Autodesk Fusion 360 part; units mm, degrees
note: some values were not read from the file. Set by a fixed rule: the direction of a hole.
(part 6 of 6)
  line L835 (112.245, -64.0081) -> (112.482, -64.0649)
  line L836 (112.482, -64.0649) -> (112.707, -64.1579)
  line L837 (112.707, -64.1579) -> (112.914, -64.285)
  line L838 (112.914, -64.285) -> (113.099, -64.443)
  line L839 (113.099, -64.443) -> (113.257, -64.6279)
  line L840 (113.257, -64.6279) -> (113.384, -64.8353)
  line L841 (113.384, -64.8353) -> (113.477, -65.06)
  line L842 (113.477, -65.06) -> (113.534, -65.2965)
  line L843 (113.534, -65.2965) -> (113.553, -65.539)
  line L844 (113.553, -65.539) -> (113.534, -65.7815)
  line L845 (113.534, -65.7815) -> (113.477, -66.018)
  line L846 (113.477, -66.018) -> (113.384, -66.2427)
  line L847 (113.384, -66.2427) -> (113.257, -66.4501)
  line L848 (113.257, -66.4501) -> (113.099, -66.635)
  line L849 (113.099, -66.635) -> (112.914, -66.793)
  line L850 (112.914, -66.793) -> (112.707, -66.9201)
  line L851 (112.707, -66.9201) -> (112.482, -67.0131)
  line L852 (112.482, -67.0131) -> (112.245, -67.0699)
  line L853 (112.245, -67.0699) -> (112.003, -67.089)
  line L854 (112.003, -67.089) -> (111.761, -67.0699)
  line L855 (111.761, -67.0699) -> (111.524, -67.0131)
  line L856 (111.524, -67.0131) -> (111.299, -66.9201)
  line L857 (111.299, -66.9201) -> (111.092, -66.793)
  line L858 (111.092, -66.793) -> (110.907, -66.635)
  line L859 (110.907, -66.635) -> (110.749, -66.4501)
  line L860 (110.749, -66.4501) -> (110.622, -66.2427)
  line L861 (110.622, -66.2427) -> (110.529, -66.018)
  line L862 (110.529, -66.018) -> (110.472, -65.7815)
  line L863 (110.472, -65.7815) -> (110.453, -65.539)
  line L864 (110.453, -65.539) -> (110.456, -65.5035)
  line L865 (110.456, -65.5035) -> (110.472, -65.2965)
  line L866 (110.472, -65.2965) -> (110.529, -65.06)
  line L867 (110.615, -65.9741) -> (110.704, -66.195)
  line L868 (110.704, -66.195) -> (110.829, -66.3983)
  line L869 (110.829, -66.3983) -> (110.985, -66.5785)
  line L870 (110.985, -66.5785) -> (111.168, -66.7308)
  line L871 (111.168, -66.7308) -> (111.374, -66.8511)
  line L872 (111.374, -66.8511) -> (111.597, -66.9362)
  line L873 (111.597, -66.9362) -> (111.831, -66.9837)
  line L874 (111.831, -66.9837) -> (112.069, -66.9925)
  line L875 (112.069, -66.9925) -> (112.306, -66.9622)
  line L876 (112.306, -66.9622) -> (112.534, -66.8937)
  line L877 (112.534, -66.8937) -> (112.748, -66.7888)
  line L878 (112.748, -66.7888) -> (112.942, -66.6503)
  line L879 (112.942, -66.6503) -> (113.111, -66.482)
  line L880 (113.111, -66.482) -> (113.25, -66.2884)
  line L881 (113.25, -66.2884) -> (113.356, -66.0746)
  line L882 (113.356, -66.0746) -> (113.425, -65.8465)
  line L883 (113.425, -65.8465) -> (113.456, -65.6101)
  line L884 (113.456, -65.6101) -> (113.458, -65.539)
  line L885 (113.458, -65.539) -> (113.438, -65.3014)
  line L886 (113.438, -65.3014) -> (113.38, -65.0701)
  line L887 (113.38, -65.0701) -> (113.285, -64.8515)
  line L888 (113.285, -64.8515) -> (113.156, -64.6513)
  line L889 (113.156, -64.6513) -> (112.995, -64.4749)
  line L890 (112.995, -64.4749) -> (112.808, -64.3271)
  line L891 (112.808, -64.3271) -> (112.599, -64.2119)
  line L892 (112.599, -64.2119) -> (112.375, -64.1323)
  line L893 (112.375, -64.1323) -> (112.14, -64.0905)
  line L894 (112.14, -64.0905) -> (111.902, -64.0876)
  line L895 (111.902, -64.0876) -> (111.666, -64.1236)
  line L896 (111.666, -64.1236) -> (111.439, -64.1977)
  line L897 (111.439, -64.1977) -> (111.228, -64.3078)
  line L898 (111.228, -64.3078) -> (111.037, -64.451)
  line L899 (111.037, -64.451) -> (110.872, -64.6234)
  line L900 (110.872, -64.6234) -> (110.738, -64.8203)
  line L901 (110.738, -64.8203) -> (110.638, -65.0366)
  line L902 (110.638, -65.0366) -> (110.574, -65.2664)
  line L903 (110.574, -65.2664) -> (110.548, -65.5035)
  line L904 (110.548, -65.5035) -> (110.562, -65.7415)
  line L905 (110.562, -65.7415) -> (110.615, -65.9741)
  line L906 (39.4089, -65.06) -> (39.5019, -64.8353)
  line L907 (39.5019, -64.8353) -> (39.629, -64.6279)
  line L908 (39.629, -64.6279) -> (39.787, -64.443)
  line L909 (39.787, -64.443) -> (39.9719, -64.285)
  line L910 (39.9719, -64.285) -> (40.1793, -64.1579)
  line L911 (40.1793, -64.1579) -> (40.404, -64.0649)
  line L912 (40.404, -64.0649) -> (40.6405, -64.0081)
  line L913 (40.6405, -64.0081) -> (40.883, -63.989)
  line L914 (40.883, -63.989) -> (41.1255, -64.0081)
  line L915 (41.1255, -64.0081) -> (41.362, -64.0649)
  line L916 (41.362, -64.0649) -> (41.5867, -64.1579)
  line L917 (41.5867, -64.1579) -> (41.7941, -64.285)
  line L918 (41.7941, -64.285) -> (41.979, -64.443)
  line L919 (41.979, -64.443) -> (42.137, -64.6279)
  line L920 (42.137, -64.6279) -> (42.2641, -64.8353)
  line L921 (42.2641, -64.8353) -> (42.3571, -65.06)
  line L922 (42.3571, -65.06) -> (42.4139, -65.2965)
  line L923 (42.4139, -65.2965) -> (42.433, -65.539)
  line L924 (42.433, -65.539) -> (42.4139, -65.7815)
  line L925 (42.4139, -65.7815) -> (42.3571, -66.018)
  line L926 (42.3571, -66.018) -> (42.2641, -66.2427)
  line L927 (42.2641, -66.2427) -> (42.137, -66.4501)
  line L928 (42.137, -66.4501) -> (41.979, -66.635)
  line L929 (41.979, -66.635) -> (41.7941, -66.793)
  line L930 (41.7941, -66.793) -> (41.5867, -66.9201)
  line L931 (41.5867, -66.9201) -> (41.362, -67.0131)
  line L932 (41.362, -67.0131) -> (41.1255, -67.0699)
  line L933 (41.1255, -67.0699) -> (40.883, -67.089)
  line L934 (40.883, -67.089) -> (40.6405, -67.0699)
  line L935 (40.6405, -67.0699) -> (40.404, -67.0131)
  line L936 (40.404, -67.0131) -> (40.1793, -66.9201)
  line L937 (40.1793, -66.9201) -> (39.9719, -66.793)
  line L938 (39.9719, -66.793) -> (39.787, -66.635)
  line L939 (39.787, -66.635) -> (39.629, -66.4501)
  line L940 (39.629, -66.4501) -> (39.5019, -66.2427)
  line L941 (39.5019, -66.2427) -> (39.4089, -66.018)
  line L942 (39.4089, -66.018) -> (39.3521, -65.7815)
  line L943 (39.3521, -65.7815) -> (39.333, -65.539)
  line L944 (39.333, -65.539) -> (39.3358, -65.5035)
  line L945 (39.3358, -65.5035) -> (39.3521, -65.2965)
  line L946 (39.3521, -65.2965) -> (39.4089, -65.06)
  line L947 (39.4946, -65.9741) -> (39.5843, -66.195)
  line L948 (39.5843, -66.195) -> (39.7089, -66.3983)
  line L949 (39.7089, -66.3983) -> (39.865, -66.5785)
  line L950 (39.865, -66.5785) -> (40.0485, -66.7308)
  line L951 (40.0485, -66.7308) -> (40.2543, -66.8511)
  line L952 (40.2543, -66.8511) -> (40.4771, -66.9362)
  line L953 (40.4771, -66.9362) -> (40.7107, -66.9837)
  line L954 (40.7107, -66.9837) -> (40.949, -66.9925)
  line L955 (40.949, -66.9925) -> (41.1855, -66.9622)
  line L956 (41.1855, -66.9622) -> (41.4139, -66.8937)
  line L957 (41.4139, -66.8937) -> (41.628, -66.7888)
  line L958 (41.628, -66.7888) -> (41.8221, -66.6503)
  line L959 (41.8221, -66.6503) -> (41.991, -66.482)
  line L960 (41.991, -66.482) -> (42.1302, -66.2884)
  line L961 (42.1302, -66.2884) -> (42.2358, -66.0746)
  line L962 (42.2358, -66.0746) -> (42.3051, -65.8465)
  line L963 (42.3051, -65.8465) -> (42.3362, -65.6101)
  line L964 (42.3362, -65.6101) -> (42.338, -65.539)
  line L965 (42.338, -65.539) -> (42.3184, -65.3014)
  line L966 (42.3184, -65.3014) -> (42.2603, -65.0701)
  line L967 (42.2603, -65.0701) -> (42.1653, -64.8515)
  line L968 (42.1653, -64.8515) -> (42.0358, -64.6513)
  line L969 (42.0358, -64.6513) -> (41.8753, -64.4749)
  line L970 (41.8753, -64.4749) -> (41.6882, -64.3271)
  line L971 (41.6882, -64.3271) -> (41.4794, -64.2119)
  line L972 (41.4794, -64.2119) -> (41.2547, -64.1323)
  line L973 (41.2547, -64.1323) -> (41.0199, -64.0905)
  line L974 (41.0199, -64.0905) -> (40.7815, -64.0876)
  line L975 (40.7815, -64.0876) -> (40.5458, -64.1236)
  line L976 (40.5458, -64.1236) -> (40.3192, -64.1977)
  line L977 (40.3192, -64.1977) -> (40.1077, -64.3078)
  line L978 (40.1077, -64.3078) -> (39.917, -64.451)
  line L979 (39.917, -64.451) -> (39.7523, -64.6234)
  line L980 (39.7523, -64.6234) -> (39.6179, -64.8203)
  line L981 (39.6179, -64.8203) -> (39.5175, -65.0366)
  line L982 (39.5175, -65.0366) -> (39.4538, -65.2664)
  line L983 (39.4538, -65.2664) -> (39.4285, -65.5035)
  line L984 (39.4285, -65.5035) -> (39.4422, -65.7415)
  line L985 (39.4422, -65.7415) -> (39.4946, -65.9741)
extrude "Extrude1" add sketch "SOLDERBREAD02_DXF_Outline_in_MilliMeters" along normal blind 2.54 contours L411 L412 L413 L414 L415 L416 L417 L418 L419 L420 L421 L422 L423 L424 L425 L426 L427 L428 L429 L430 L433 L434 L435 L436 L437 L440 L443 L444 L445 L446 L447 L450 L451 L452 L453 L454 L455 L456 L457 L458 L459 L460 L461 L462 L463 L464 L465 L466 L467 L468 L469 L470 L471 L472 L473 L474 L475 L476 L477 L478 L479 L480 L481 L482 L483 L484 L485 L486 L487 L488 L489 L490 L491 L492 L493 L494 L495 L496 L497 L498 L499 L500 L501 L502 L503 L504 L505 L506 L507 L508 L509 L510 L511 L512 L513 L514 L515 L516 L517 L518 L519 L520 L521 L523 L524 L525 L526 L527 L528 L529 L532 L533 L534 L535 L536 L537 L538 L539 L540 L541 L542 L543 L544 L545 L546 L547 L548 L549 L550 L551 L552 L553 L554 L555 L556 L557 L558 L559 L560 L561 L562 L563 L564 L565 L566 L567 L568 L569 L570 L571 L572 L573 L574 L575 L576 L577 L578 L579 L580 L581 L582 L583 L584 L585 L586 L587 L588 L589 L590 L591 L592 L593 L594 L595 L596 L599 L600 L601 L602 L603 L604 L605 L608 L609 L610 L611 L612 L616 L617 L618 L619 L620 L621 L622 L623 L624 L625 L626 L627 L628 L629 L630 L631 L632 L633 L634 L635 L636 L637 L638 L639 L640 L641 L642 L643 L644 L645 L646 L647 L648 L649 L650 L651 L652 L653 L654 L655 L656 L657 L658 L659 L660 L661 L662 L663 L664 L665 L666 L667 L668 L669 L670 L671 L672 L673 L674 L675 L676 L677 L678 L679 L680 L681 L682 L684 L685 L686 L687 L688 L689 L690 L691 L692 L693 L694 L695 L696 L697 L700 L701 L702 L703 L704 L705 L706 L707 L708 L709 L710 L711 L712 L713 L714 L715 L716 L717 L718 L719 L720 L721 L722 L723 L724 L725 L726 L727 L728 L729 L730 L731 L732 L733 L734 L735 L736 L737 L738 L739 L740 L741 L742 L743 L744 L745

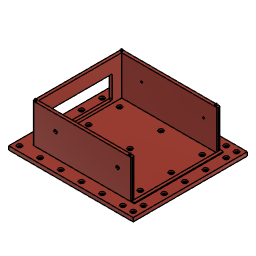
design "base"
Autodesk Fusion 360 part; units mm, degrees
sketch "Sketch1" plane through (0, 0, 0) normal (0, 0, 1) x (1, 0, 0)
  line L0 (0, 0) -> (232, 0)
  line L1 (232, 0) -> (232, 201)
  line L2 (232, 201) -> (0, 201)
  line L3 (0, 201) -> (0, 0)
  line L4 (0, 201) -> (-7, 201)
  line L5 (0, 201) -> (-7, 201)
  line L6 (-7, 201) -> (-7, 208)
  line L7 (-7, 208) -> (0, 208)
  line L8 (0, 208) -> (0, 201)
  line L9 (232, 0) -> (239, 0)
  line L10 (239, 0) -> (239, -7)
  line L11 (239, -7) -> (232, -7)
  line L12 (232, -7) -> (232, 0)
  line L13 (-7, 208) -> (239, 208)
  line L14 (239, 208) -> (239, -7)
  line L15 (239, -7) -> (-7, -7)
  line L16 (-7, -7) -> (-7, 208)
  line L17 (232, 201) -> (232, 208)
  line L18 (239, 208) -> (239, 240.3287)
  line L19 (-21.5407, 238.3287) -> (-21.5407, 225.3287)
  line L20 (-21.5407, 225.3287) -> (-34.5407, 225.3287)
  circle A0 centre (-21.5407, -24.6713) radius 5.75
  line L21 (266.4593, -37.6713) -> (253.4593, -37.6713)
  circle A1 centre (-21.5407, 25.3287) radius 3
  line L22 (253.4593, -37.6713) -> (253.4593, -24.6713)
  circle A2 centre (-21.5407, 225.3287) radius 5.75
  line L23 (-34.5407, 238.3287) -> (-21.5407, 238.3287)
  line L24 (-34.5407, 225.3287) -> (-34.5407, 238.3287)
  line L25 (253.4593, -24.6713) -> (266.4593, -24.6713)
  circle A3 centre (28.4593, -24.6713) radius 3
  circle A4 centre (-21.5407, 225.3287) radius 3
  circle A5 centre (253.4593, 0.3287) radius 5.75
  line L26 (266.4593, -24.6713) -> (266.4593, -37.6713)
  circle A6 centre (253.4593, -24.6713) radius 5.75
  circle A7 centre (-21.5407, 25.3287) radius 5.75
  circle A8 centre (253.4593, -24.6713) radius 3
  circle A9 centre (-21.5407, 75.3287) radius 3
  circle A10 centre (253.4593, 0.3287) radius 3
  circle A11 centre (253.4593, 50.3287) radius 5.75
  circle A12 centre (253.4593, 50.3287) radius 3
  circle A13 centre (128.4593, -24.6713) radius 5.75
  circle A14 centre (78.4593, -24.6713) radius 3
  circle A15 centre (28.4593, 225.3287) radius 3
  circle A16 centre (-21.5407, -24.6713) radius 3
  circle A17 centre (228.4593, -24.6713) radius 3
  circle A18 centre (78.4593, -24.6713) radius 5.75
  circle A19 centre (253.4593, 225.3287) radius 3
  circle A20 centre (253.4593, 225.3287) radius 5.75
  circle A21 centre (-21.5407, 175.3287) radius 3
  circle A22 centre (-21.5407, 125.3287) radius 3
  circle A23 centre (-21.5407, 125.3287) radius 5.75
  circle A24 centre (28.4593, -24.6713) radius 5.75
  circle A25 centre (-21.5407, 175.3287) radius 5.75
  line L27 (232.8, 201) -> (232.8, 208)
  circle A26 centre (78.4593, 225.3287) radius 3
  circle A27 centre (178.4593, 225.3287) radius 5.75
  circle A28 centre (128.4593, 225.3287) radius 5.75
  circle A29 centre (178.4593, 225.3287) radius 3
  circle A30 centre (178.4593, -24.6713) radius 3
  circle A31 centre (128.4593, -24.6713) radius 3
  circle A32 centre (28.4593, 225.3287) radius 5.75
  circle A33 centre (228.4593, 225.3287) radius 5.75
  circle A34 centre (253.4593, 200.3287) radius 3
  line L28 (266.4593, 238.3287) -> (266.4593, -37.6713)
  circle A35 centre (128.4593, 225.3287) radius 3
  circle A36 centre (-21.5407, 75.3287) radius 5.75
  circle A37 centre (228.4593, 225.3287) radius 3
  line L29 (266.4593, -37.6713) -> (-34.5407, -37.6713)
  line L30 (-34.5407, -37.6713) -> (-34.5407, 238.3287)
  circle A38 centre (228.4593, -24.6713) radius 5.75
  circle A39 centre (78.4593, 225.3287) radius 5.75
  circle A40 centre (178.4593, -24.6713) radius 5.75
  circle A41 centre (253.4593, 200.3287) radius 5.75
  line L31 (-34.5407, 238.3287) -> (266.4593, 238.3287)
  circle A42 centre (253.4593, 100.3287) radius 5.75
  circle A43 centre (253.4593, 150.3287) radius 3
  circle A44 centre (253.4593, 100.3287) radius 3
  circle A45 centre (253.4593, 150.3287) radius 5.75
  circle A46 centre (16, 180) radius 3.375
  circle A47 centre (16, 180) radius 5.75
  circle A48 centre (116, 180) radius 3.375
  circle A49 centre (116, 180) radius 5.75
  circle A50 centre (216, 180) radius 3.375
  circle A51 centre (216, 180) radius 5.75
  circle A52 centre (16, 105) radius 3.375
  circle A53 centre (16, 105) radius 5.75
  circle A54 centre (116, 105) radius 3.375
  circle A55 centre (116, 105) radius 5.75
  circle A56 centre (216, 105) radius 3.375
  circle A57 centre (216, 105) radius 5.75
  circle A58 centre (16, 30) radius 3.375
  circle A59 centre (16, 30) radius 5.75
  circle A60 centre (116, 30) radius 3.375
  circle A61 centre (116, 30) radius 5.75
  circle A62 centre (216, 30) radius 3.375
  circle A63 centre (216, 30) radius 5.75
  point P0 (0.8, 0)
  point P1 (0.8, 0)
  point P2 (0.8, 0)
  dimension "d2" = 201
  dimension "d3" = 7
  dimension "d4" = 7
  dimension "d5" = 7
  dimension "d6" = 7
  dimension "d56" = 7
  dimension "d156" = 25
  dimension "d157" = -25
  dimension "d160" = 25
  dimension "d161" = -25
  dimension "d162" = 11.5
  dimension "d163" = 6
  dimension "d164" = 13
  dimension "d165" = 13
  dimension "d166" = 13
  dimension "d167" = 13
  dimension "d168" = 7
  dimension "d223" = 6.75
  dimension "d224" = 11.5
  dimension "d227" = 100
  dimension "d228" = -75
  constraint vertical L1
  constraint horizontal L2
  constraint vertical L3
  constraint coincident L0.start L3.end
  constraint perpendicular L3 L4
  constraint horizontal L5
  constraint vertical L6
  constraint horizontal L7
  constraint vertical L8
  constraint horizontal L13
  constraint vertical L14
  constraint vertical L16
  constraint perpendicular L13 L17
  constraint concentric A2 A4
  constraint horizontal L20
  constraint vertical L24
  constraint horizontal L23
  constraint vertical L19
  constraint coincident L19.end L20.start
  constraint horizontal L25
  constraint vertical L26
  constraint horizontal L21
  constraint vertical L22
  constraint coincident L22.end L25.start
  constraint horizontal L29
  constraint vertical L30
  constraint horizontal L31
  constraint vertical L28
  constraint concentric A46 A47
  measures "d2" distance of L0.start L2.end
  measures "d3" distance of L2.end L4.end
  measures "d4" distance of L2.end L4.end
  measures "d5" distance of L2.end L7.end
  measures "d6" distance of L0.end L9.end
  measures "d56" distance of L1.end L17.end
  measures "d162" diameter of A2
  measures "d163" diameter of A4
  measures "d164" distance of L19.end L20.end
  measures "d165" distance of L19.end L19.start
  measures "d166" distance of L22.end L25.end
  measures "d167" distance of L22.end L21.end
  measures "d168" distance of L27.end L27.start
  measures "d223" diameter of A46
  measures "d224" diameter of A47
sketch "Sketch2" plane through (0, 0, 0) normal (0, 0, 1) x (1, 0, 0)
  circle A0 centre (-22.3407, 225.3287) radius 5.75
  circle A1 centre (27.6593, 225.3287) radius 5.75
  circle A2 centre (77.6593, 225.3287) radius 5.75
  circle A3 centre (127.6593, 225.3287) radius 5.75
  circle A4 centre (177.6593, 225.3287) radius 5.75
  circle A5 centre (227.6593, 225.3287) radius 5.75
  circle A6 centre (252.6593, 225.3287) radius 5.75
  circle A7 centre (252.6593, 200.3287) radius 5.75
  circle A8 centre (-22.3407, 175.3287) radius 5.75
  circle A9 centre (252.6593, 150.3287) radius 5.75
  circle A10 centre (-22.3407, 125.3287) radius 5.75
  circle A11 centre (252.6593, 100.3287) radius 5.75
  circle A12 centre (-22.3407, 75.3287) radius 5.75
  circle A13 centre (252.6593, 50.3287) radius 5.75
  circle A14 centre (-22.3407, 25.3287) radius 5.75
  circle A15 centre (252.6593, 0.3287) radius 5.75
  circle A16 centre (-22.3407, -24.6713) radius 5.75
  circle A17 centre (27.6593, -24.6713) radius 5.75
  circle A18 centre (77.6593, -24.6713) radius 5.75
  circle A19 centre (127.6593, -24.6713) radius 5.75
  circle A20 centre (177.6593, -24.6713) radius 5.75
  circle A21 centre (227.6593, -24.6713) radius 5.75
  circle A22 centre (252.6593, -24.6713) radius 5.75
  circle A23 centre (-22.3407, 225.3287) radius 3
  circle A24 centre (27.6593, 225.3287) radius 3
  circle A25 centre (77.6593, 225.3287) radius 3
  circle A26 centre (127.6593, 225.3287) radius 3
  circle A27 centre (177.6593, 225.3287) radius 3
  circle A28 centre (227.6593, 225.3287) radius 3
  circle A29 centre (252.6593, 225.3287) radius 3
  circle A30 centre (252.6593, 200.3287) radius 3
  circle A31 centre (-22.3407, 175.3287) radius 3
  circle A32 centre (252.6593, 150.3287) radius 3
  circle A33 centre (-22.3407, 125.3287) radius 3
  circle A34 centre (252.6593, 100.3287) radius 3
  circle A35 centre (-22.3407, 75.3287) radius 3
  circle A36 centre (252.6593, 50.3287) radius 3
  circle A37 centre (-22.3407, 25.3287) radius 3
  circle A38 centre (252.6593, 0.3287) radius 3
  circle A39 centre (-22.3407, -24.6713) radius 3
  circle A40 centre (27.6593, -24.6713) radius 3
  circle A41 centre (77.6593, -24.6713) radius 3
  circle A42 centre (127.6593, -24.6713) radius 3
  circle A43 centre (177.6593, -24.6713) radius 3
  circle A44 centre (227.6593, -24.6713) radius 3
  circle A45 centre (252.6593, -24.6713) radius 3
  line L0 (-22.3407, 225.3287) -> (-35.3407, 225.3287)
  line L1 (-35.3407, 225.3287) -> (-35.3407, 238.3287)
  line L2 (-35.3407, 238.3287) -> (-22.3407, 238.3287)
  line L3 (-22.3407, 238.3287) -> (-22.3407, 225.3287)
  line L4 (252.6593, -24.6713) -> (265.6593, -24.6713)
  line L5 (265.6593, -24.6713) -> (265.6593, -37.6713)
  line L6 (265.6593, -37.6713) -> (252.6593, -37.6713)
  line L7 (252.6593, -37.6713) -> (252.6593, -24.6713)
  line L8 (265.6593, -37.6713) -> (-35.3407, -37.6713)
  line L9 (-35.3407, -37.6713) -> (-35.3407, 238.3287)
  line L10 (-35.3407, 238.3287) -> (265.6593, 238.3287)
  line L11 (265.6593, 238.3287) -> (265.6593, -37.6713)
  line L12 (232, 201) -> (232, 208)
  dimension "d8" = 11.5
  dimension "d11" = 25
  dimension "d12" = -25
  dimension "d13" = 6
  dimension "d16" = 25
  dimension "d17" = -25
  dimension "d18" = 13
  dimension "d19" = 13
  dimension "d20" = 13
  dimension "d21" = 13
  dimension "d153" = 7
  constraint concentric A0 A23
  constraint horizontal L0
  constraint vertical L1
  constraint horizontal L2
  constraint vertical L3
  constraint coincident A0.centre A23.centre
  constraint horizontal L4
  constraint vertical L5
  constraint horizontal L6
  constraint vertical L7
  constraint coincident A22.centre A45.centre
  constraint horizontal L8
  constraint vertical L9
  constraint horizontal L10
  constraint vertical L11
  measures "d8" diameter of A0
  measures "d13" diameter of A23
  measures "d18" distance of A0.centre L0.end
  measures "d19" distance of A0.centre L2.end
  measures "d20" distance of A22.centre L4.end
  measures "d21" distance of A22.centre L6.end
  measures "d153" distance of L12.start L12.end
extrude "Extrude3" add sketch "Sketch1" along normal blind 7 contours L0 L1 L2 L3 | L0 L3 L4 L5 L12 L15 L16 | L1 L9 L13 L14 L17 | L9 L10 L11 L12 L14 L15 | L2 L8 L13 L17 | L4 L5 L6 L7 L8 L13 L16 makes body 1
extrude "Extrude4" add sketch "Sketch1" along normal blind 102 contours L0 L3 L4 L5 L12 L15 L16 | L2 L8 L13 L17 | L4 L5 L6 L7 L8 L13 L16 bodies 1
sketch "Sketch4" plane through (0, 0, 102) normal (0, 0, 1) x (-1, 0, 0)
  line L0 (0, -201) -> (-232, -201)
  line L1 (-232, -201) -> (-232, -208)
  line L2 (-232, -208) -> (7, -208)
  line L3 (7, -208) -> (7, 7)
  line L4 (7, 7) -> (-232, 7)
  line L5 (-232, 0) -> (0, 0)
  line L6 (0, 0) -> (0, -201)
  line L7 (7, -208) -> (-232, -208)
  line L8 (-232, -208) -> (-232, 0)
  line L9 (-232, 0) -> (7, 0)
  line L10 (7, 0) -> (7, -208)
  line L11 (-36, -158) -> (-198, -158)
  line L12 (-198, -158) -> (-198, -43)
  line L13 (-198, -43) -> (-36, -43)
  line L14 (-36, -43) -> (-36, -158)
  line L15 (7, -208) -> (-232, -208)
  line L16 (-232, -208) -> (-232, 7)
  line L17 (-232, 7) -> (7, 7)
  line L18 (7, 7) -> (7, -208)
  line L19 (-232, 7) -> (-225, 7)
  line L20 (-225, 7) -> (-225, 3.5)
  line L21 (-225, 3.5) -> (-232, 3.5)
  line L22 (-232, 3.5) -> (-232, 7)
  line L23 (7, 7) -> (3.5, 7)
  line L24 (3.5, 7) -> (3.5, 3.5)
  line L25 (3.5, 3.5) -> (7, 3.5)
  line L26 (7, 3.5) -> (7, 7)
  line L27 (7, -208) -> (3.5, -208)
  line L28 (3.5, -208) -> (3.5, -204.5)
  line L29 (3.5, -204.5) -> (7, -204.5)
  line L30 (7, -204.5) -> (7, -208)
  line L31 (-232, -208) -> (-225, -208)
  line L32 (-225, -208) -> (-225, -204.5)
  line L33 (-225, -204.5) -> (-232, -204.5)
  line L34 (-232, -204.5) -> (-232, -208)
  line L35 (1.625, -202.625) -> (5.375, -202.625)
  line L36 (5.375, -202.625) -> (5.375, -206.375)
  line L37 (5.375, -206.375) -> (1.625, -206.375)
  line L38 (1.625, -206.375) -> (1.625, -202.625)
  line L39 (1.625, -202.625) -> (5.375, -206.375) construction
  line L40 (5.375, -202.625) -> (1.625, -206.375) construction
  line L41 (1.625, 5.375) -> (5.375, 5.375)
  line L42 (5.375, 5.375) -> (5.375, 1.625)
  line L43 (5.375, 1.625) -> (1.625, 1.625)
  line L44 (1.625, 1.625) -> (1.625, 5.375)
  line L45 (1.625, 5.375) -> (5.375, 1.625) construction
  line L46 (5.375, 5.375) -> (1.625, 1.625) construction
  line L47 (-226.875, 5.375) -> (-223.125, 5.375)
  line L48 (-223.125, 5.375) -> (-223.125, 1.625)
  line L49 (-223.125, 1.625) -> (-226.875, 1.625)
  line L50 (-226.875, 1.625) -> (-226.875, 5.375)
  line L51 (-226.875, 5.375) -> (-223.125, 1.625) construction
  line L52 (-223.125, 5.375) -> (-226.875, 1.625) construction
  line L53 (-226.875, -202.625) -> (-223.125, -202.625)
  line L54 (-223.125, -202.625) -> (-223.125, -206.375)
  line L55 (-223.125, -206.375) -> (-226.875, -206.375)
  line L56 (-226.875, -206.375) -> (-226.875, -202.625)
  line L57 (-226.875, -202.625) -> (-223.125, -206.375) construction
  line L58 (-223.125, -202.625) -> (-226.875, -206.375) construction
  line L59 (-36, -158) -> (-15.2, -158)
  line L60 (-15.2, -158) -> (-15.2, -179.35)
  line L61 (-15.2, -179.35) -> (-36, -179.35)
  line L62 (-36, -179.35) -> (-36, -158)
  line L63 (-198, -43) -> (-218.8, -43)
  line L64 (-218.8, -43) -> (-218.8, -21.65)
  line L65 (-218.8, -21.65) -> (-198, -21.65)
  line L66 (-198, -21.65) -> (-198, -43)
  line L67 (-15.2, -179.35) -> (-218.8, -179.35)
  line L68 (-218.8, -179.35) -> (-218.8, -21.65)
  line L69 (-218.8, -21.65) -> (-15.2, -21.65)
  line L70 (-15.2, -21.65) -> (-15.2, -179.35)
  line L71 (-15.2, -179.35) -> (-10.2, -179.35)
  line L72 (-10.2, -179.35) -> (-10.2, -184.35)
  line L73 (-10.2, -184.35) -> (-15.2, -184.35)
  line L74 (-15.2, -184.35) -> (-15.2, -179.35)
  line L75 (-218.8, -21.65) -> (-223.8, -21.65)
  line L76 (-223.8, -21.65) -> (-223.8, -16.65)
  line L77 (-223.8, -16.65) -> (-218.8, -16.65)
  line L78 (-218.8, -16.65) -> (-218.8, -21.65)
  line L79 (-10.2, -184.35) -> (-223.8, -184.35)
  line L80 (-223.8, -184.35) -> (-223.8, -16.65)
  line L81 (-223.8, -16.65) -> (-10.2, -16.65)
  line L82 (-10.2, -16.65) -> (-10.2, -184.35)
  line L83 (-232, 7) -> (-232, 0)
  point P0 (3.5, -204.5)
  point P1 (3.5, 3.5)
  point P2 (-225, 3.5)
  point P3 (-225, -204.5)
  dimension "d59" = 162
  dimension "d60" = 115
  dimension "d89" = 7
  dimension "d90" = 3.5
  dimension "d91" = 3.5
  dimension "d92" = 3.5
  dimension "d93" = 3.5
  dimension "d94" = 3.5
  dimension "d95" = 7
  dimension "d96" = 3.75
  dimension "d97" = 3.75
  dimension "d98" = 3.75
  dimension "d99" = 3.75
  dimension "d100" = 3.75
  dimension "d101" = 3.75
  dimension "d102" = 3.75
  dimension "d103" = 3.75
  dimension "d104" = 20.8
  dimension "d105" = 21.35
  dimension "d106" = 20.8
  dimension "d107" = 21.35
  dimension "d108" = 5
  dimension "d109" = 5
  dimension "d110" = 5
  dimension "d111" = 5
  dimension "d112" = 3.5
  constraint horizontal L7
  constraint vertical L8
  constraint horizontal L9
  constraint vertical L10
  constraint coincident L5.start L8.end
  constraint coincident L2.end L3.start
  constraint horizontal L11
  constraint vertical L12
  constraint horizontal L13
  constraint vertical L14
  constraint horizontal L15
  constraint vertical L16
  constraint horizontal L17
  constraint vertical L18
  constraint coincident L4.end L16.end
  constraint horizontal L19
  constraint vertical L20
  constraint horizontal L21
  constraint vertical L22
  constraint horizontal L23
  constraint vertical L24
  constraint horizontal L25
  constraint vertical L26
  constraint coincident L3.end L4.start
  constraint horizontal L27
  constraint vertical L28
  constraint horizontal L29
  constraint vertical L30
  constraint horizontal L31
  constraint vertical L32
  constraint horizontal L33
  constraint vertical L34
  constraint horizontal L35
  constraint perpendicular L35 L36
  constraint parallel L35 L37
  constraint parallel L36 L38
  constraint coincident L39 P0
  constraint coincident L40 P0
  constraint coincident P0 L28.end
  constraint horizontal L41
  constraint perpendicular L41 L42
  constraint parallel L41 L43
  constraint parallel L42 L44
  constraint coincident L45 P1
  constraint coincident L46 P1
  constraint coincident P1 L24.end
  constraint horizontal L47
  constraint perpendicular L47 L48
  constraint parallel L47 L49
  constraint parallel L48 L50
  constraint coincident L51 P2
  constraint coincident L52 P2
  constraint coincident P2 L20.end
  constraint horizontal L53
  constraint perpendicular L53 L54
  constraint parallel L53 L55
  constraint parallel L54 L56
  constraint coincident L57 P3
  constraint coincident L58 P3
  constraint coincident P3 L32.end
  constraint horizontal L59
  constraint vertical L60
  constraint horizontal L61
  constraint vertical L62
  constraint horizontal L63
  constraint vertical L64
  constraint horizontal L65
  constraint vertical L66
  constraint horizontal L67
  constraint vertical L68
  constraint horizontal L69
  constraint vertical L70
  constraint horizontal L71
  constraint vertical L72
  constraint horizontal L73
  constraint vertical L74
  constraint horizontal L75
  constraint vertical L76
  constraint horizontal L77
  constraint vertical L78
  constraint horizontal L79
  constraint vertical L80
  constraint horizontal L81
  constraint vertical L82
  measures "d59" distance of L11.start L11.end
  measures "d60" distance of L11.start L13.end
  measures "d89" distance of L4.end L19.end
  measures "d90" distance of L4.end L21.end
  measures "d91" distance of L3.end L23.end
  measures "d92" distance of L3.end L25.end
  measures "d93" distance of L2.end L27.end
  measures "d94" distance of L2.end L29.end
  measures "d95" distance of L1.end L31.end
  measures "d96" distance of L36.end L37.end
  measures "d97" distance of L35.end L36.end
  measures "d98" distance of L42.end L43.end
  measures "d99" distance of L41.end L42.end
  measures "d100" distance of L48.end L49.end
  measures "d101" distance of L47.end L48.end
  measures "d102" distance of L54.end L55.end
  measures "d103" distance of L53.end L54.end
  measures "d104" distance of L11.start L59.end
  measures "d105" distance of L11.start L61.end
  measures "d106" distance of L12.end L63.end
  measures "d107" distance of L12.end L65.end
  measures "d108" distance of L60.end L71.end
  measures "d109" distance of L60.end L73.end
  measures "d110" distance of L64.end L75.end
  measures "d111" distance of L64.end L77.end
  measures "d112" distance of L1.end L33.end
extrude "Extrude5" add sketch "Sketch1" along normal blind 11 contours L1 L9 L13 L14 L17 | L9 L10 L11 L12 L14 L15 bodies 1
sketch "Sketch5" plane through (0, -7, 0) normal (0, -1, 0) x (1, 0, 0)
  line L0 (-7, 0) -> (239, 0)
  line L1 (232, 11) -> (232, 102)
  line L2 (-7, 102) -> (-7, 0)
  line L3 (-7, 102) -> (15, 102)
  line L4 (0, 0) -> (0, 7)
  line L5 (15, 102) -> (232, 102)
  line L6 (232, 102) -> (232, 5.2162)
  line L7 (232, 5.2162) -> (15, 5.2162)
  line L8 (15, 5.2162) -> (15, 102)
  line L9 (0, 7) -> (48, 7)
  line L10 (48, 7) -> (48, 64.5)
  line L11 (48, 64.5) -> (0, 64.5)
  line L12 (0, 64.5) -> (0, 7)
  line L13 (48, 64.5) -> (198, 64.5)
  circle A0 centre (48, 64.5) radius 2.25
  circle A1 centre (198, 64.5) radius 2.25
  circle A2 centre (48, 64.5) radius 4
  circle A3 centre (198, 64.5) radius 4
  line L14 (232, 102) -> (-7, 102)
  line L15 (-7, 0) -> (-7, 5)
  line L16 (239, 0) -> (239, 11)
  line L17 (239, 11) -> (232, 11)
  dimension "d65" = 22
  dimension "d66" = 7
  dimension "d67" = 48
  dimension "d68" = 57.5
  dimension "d69" = 150
  dimension "d70" = 4.5
  dimension "d71" = 4.5
  dimension "d81" = 8
  dimension "d82" = 8
  constraint coincident L2.start L3.start
  constraint perpendicular L2 L3
  constraint coincident L4.start origin
  constraint perpendicular L0 L4
  constraint horizontal L5
  constraint vertical L6
  constraint horizontal L7
  constraint vertical L8
  constraint coincident L1 L6.end
  constraint horizontal L9
  constraint vertical L10
  constraint horizontal L11
  constraint vertical L12
  constraint perpendicular L10 L13
  constraint coincident L10.end L11.start
  constraint coincident L13.end A1.centre
  constraint concentric A0 A2
  constraint concentric A1 A3
  constraint coincident L0.start L2.end
  constraint coincident L2 L15.end
  constraint perpendicular L0 L15
  measures "d65" distance of L2.start L3.end
  measures "d66" distance of L4.start L4.end
  measures "d67" distance of L4.end L9.end
  measures "d68" distance of L4.end L11.end
  measures "d69" distance of L10.end L13.end
  measures "d70" diameter of A0
  measures "d71" diameter of A1
  measures "d81" diameter of A2
  measures "d82" diameter of A3
sketch "Sketch6" plane through (0, 208, 0) normal (0, 1, 0) x (-1, 0, 0)
  line L0 (-239, 0) -> (7, 0)
  line L1 (7, 0) -> (7, 102)
  line L2 (-232, 102) -> (-232, 11)
  line L3 (7, 0) -> (-15, 0)
  line L4 (-15, 0) -> (-15, 7)
  line L5 (-15, 7) -> (7, 7)
  line L6 (7, 7) -> (7, 0)
  line L7 (-15, 7) -> (-48, 7)
  line L8 (-48, 7) -> (-48, 64.5)
  line L9 (-48, 64.5) -> (-15, 64.5)
  line L10 (-15, 64.5) -> (-15, 7)
  line L11 (-48, 64.5) -> (-198, 64.5)
  circle A0 centre (-198, 64.5) radius 2.25
  circle A1 centre (-48, 64.5) radius 2.25
  circle A2 centre (-198, 64.5) radius 4
  circle A3 centre (-48, 64.5) radius 4
  line L12 (7, 102) -> (-232, 102)
  line L13 (-232, 11) -> (-239, 11)
  line L14 (-239, 11) -> (-239, 0)
  dimension "d72" = 22
  dimension "d73" = 7
  dimension "d74" = 33
  dimension "d75" = 57.5
  dimension "d76" = 150
  dimension "d77" = 4.5
  dimension "d78" = 4.5
  dimension "d83" = 8
  dimension "d84" = 8
  constraint horizontal L3
  constraint vertical L4
  constraint horizontal L5
  constraint vertical L6
  constraint coincident L0.end L1.start
  constraint horizontal L7
  constraint vertical L8
  constraint horizontal L9
  constraint vertical L10
  constraint horizontal L11
  constraint coincident L11.end A0.centre
  constraint coincident L8.end L9.start
  constraint concentric A0 A2
  constraint concentric A1 A3
  measures "d72" distance of L0.end L3.end
  measures "d73" distance of L0.end L5.end
  measures "d74" distance of L4.end L7.end
  measures "d75" distance of L4.end L9.end
  measures "d76" distance of L8.end L11.end
  measures "d77" diameter of A0
  measures "d78" diameter of A1
  measures "d83" diameter of A2
  measures "d84" diameter of A3
extrude "Extrude7" cut sketch "Sketch5" against normal blind 221 contours L11 L13 A0 | L10 L11 A0 | L10 L13 A0 | A1 bodies 1
extrude "Extrude8" cut sketch "Sketch6" against normal blind 3 contours L8 L11 A1 A3 | L8 L9 A1 A3 | L9 L11 A1 A3 | A2 bodies 1
extrude "Extrude9" cut sketch "Sketch5" against normal blind 3 contours L11 L13 A0 A2 | L10 L11 A0 A2 | L10 L13 A0 A2 | A3 bodies 1
sketch "Sketch7" plane through (0, 0, 0) normal (0, 0, 1) x (1, 0, 0)
  line L0 (632.0908, 17.9092) -> (400, 17.9092)
  line L1 (398.5, -2.5) -> (398.5, -6.5)
  line L2 (398.5, 201.5) -> (394.5, 205.5) construction
  line L3 (422.9, 178.85) -> (417.9, 178.85)
  line L4 (422.9, 183.85) -> (422.9, 178.85)
  line L5 (393, -8) -> (393, 207)
  line L6 (393, -8) -> (632, -8)
  line L7 (393, 207) -> (393, -8)
  line L8 (396.5, 207) -> (396.5, 203.5)
  line L9 (400, 17.9092) -> (400, 200)
  line L10 (393, -4.5) -> (393, -8)
  line L11 (632, 207) -> (393, 207)
  line L12 (398.5, 205.5) -> (398.5, 201.5)
  line L13 (393, 203.5) -> (393, 207)
  line L14 (632, 200) -> (632, 207)
  line L15 (394.5, 201.5) -> (394.5, 205.5)
  line L16 (396.5, -8) -> (396.5, -4.5)
  line L17 (417.9, 178.85) -> (417.9, 183.85)
  line L18 (632, -8) -> (632.0908, 17.9092)
  line L19 (394.5, -6.5) -> (398.5, -2.5) construction
  line L20 (394.5, -6.5) -> (394.5, -2.5)
  line L21 (394.5, 201.5) -> (398.5, 205.5) construction
  line L22 (400, 200) -> (632, 200)
  line L23 (396.5, -4.5) -> (393, -4.5)
  line L24 (393, 207) -> (632, 207)
  line L25 (625, 207) -> (625, 203.5)
  line L26 (627, -6.5) -> (623, -2.5) construction
  line L27 (623, -6.5) -> (623, -2.5)
  line L28 (632, 207) -> (625, 207)
  line L29 (623, -6.5) -> (627, -2.5) construction
  line L30 (623, 201.5) -> (627, 205.5) construction
  line L31 (632, 207) -> (632, -8)
  line L32 (625, -4.5) -> (632, -4.5)
  line L33 (623, -2.5) -> (627, -2.5)
  line L34 (627, -6.5) -> (623, -6.5)
  line L35 (627, -2.5) -> (627, -6.5)
  line L36 (627, 201.5) -> (623, 205.5) construction
  line L37 (632, -4.5) -> (632, -8)
  line L38 (398.5, -6.5) -> (394.5, -2.5) construction
  line L39 (393, 207) -> (396.5, 207)
  line L40 (398.5, -6.5) -> (394.5, -6.5)
  line L41 (394.5, 205.5) -> (398.5, 205.5)
  line L42 (417.9, 183.85) -> (422.9, 183.85)
  line L43 (394.5, -2.5) -> (398.5, -2.5)
  line L44 (632, -8) -> (393, -8)
  line L45 (393, -1) -> (393, 207)
  line L46 (393, -8) -> (396.5, -8)
  line L47 (632.0908, 17.9092) -> (393, -1)
  line L48 (627, 205.5) -> (627, 201.5)
  line L49 (632, 203.5) -> (632, 207)
  line L50 (631.5, 16.15) -> (626.5, 16.15)
  line L51 (632, -8) -> (625, -8)
  line L52 (625, 203.5) -> (632, 203.5)
  line L53 (625, -8) -> (625, -4.5)
  line L54 (398.5, 201.5) -> (394.5, 201.5)
  line L55 (631.5, 21.15) -> (631.5, 16.15)
  line L56 (632, 207) -> (632.0908, 17.9092)
  line L57 (393, 207) -> (632, 207)
  line L58 (623, 201.5) -> (623, 205.5)
  line L59 (623, 205.5) -> (627, 205.5)
  line L60 (627, 201.5) -> (623, 201.5)
  line L61 (396.5, 203.5) -> (393, 203.5)
  line L62 (627, 178.85) -> (632, 178.85)
  line L63 (632, 178.85) -> (632, 183.85)
  line L64 (632, 183.85) -> (627, 183.85)
  line L65 (627, 183.85) -> (627, 178.85)
  line L66 (417.9, 183.85) -> (632, 183.85)
  line L67 (632, 183.85) -> (632, 15.15)
  line L68 (632, 15.15) -> (417.9, 15.15)
  line L69 (417.9, 15.15) -> (417.9, 183.85)
  line L70 (417.9, 15.15) -> (422.9, 15.15)
  line L71 (422.9, 15.15) -> (422.9, 20.15)
  line L72 (422.9, 20.15) -> (417.9, 20.15)
  line L73 (417.9, 20.15) -> (417.9, 15.15)
  line L74 (632, 15.15) -> (627, 15.15)
  line L75 (627, 15.15) -> (627, 20.15)
  line L76 (627, 20.15) -> (632, 20.15)
  line L77 (632, 20.15) -> (632, 15.15)
  line L78 (627, 20.15) -> (422.9, 20.15)
  line L79 (422.9, 20.15) -> (422.9, 178.85)
  line L80 (422.9, 178.85) -> (627, 178.85)
  line L81 (627, 178.85) -> (627, 20.15)
  line L82 (422.9, 178.85) -> (447.9, 178.85)
  line L83 (447.9, 178.85) -> (447.9, 155.85)
  line L84 (447.9, 155.85) -> (422.9, 155.85)
  line L85 (422.9, 155.85) -> (422.9, 178.85)
  line L86 (627, 20.15) -> (602, 20.15)
  line L87 (602, 20.15) -> (602, 43.15)
  line L88 (602, 43.15) -> (627, 43.15)
  line L89 (627, 43.15) -> (627, 20.15)
  line L90 (447.9, 155.85) -> (602, 155.85)
  line L91 (602, 155.85) -> (602, 43.15)
  line L92 (602, 43.15) -> (447.9, 43.15)
  line L93 (447.9, 43.15) -> (447.9, 155.85)
  point P0 (396.5, 203.5)
  point P1 (625, -4.5)
  point P2 (625, 203.5)
  point P3 (400, -1)
  point P4 (396.5, -4.5)
  dimension "d115" = 7
  dimension "d116" = 3.5
  dimension "d117" = 3.5
  dimension "d118" = 3.5
  dimension "d119" = 3.5
  dimension "d120" = 3.5
  dimension "d121" = 7
  dimension "d122" = 4
  dimension "d123" = 4
  dimension "d124" = 4
  dimension "d125" = 4
  dimension "d126" = 4
  dimension "d127" = 4
  dimension "d128" = 4
  dimension "d129" = 4
  dimension "d134" = 5
  dimension "d135" = 5
  dimension "d138" = 3.5
  dimension "d147" = 204.1
  dimension "d188" = 5
  dimension "d189" = 5
  dimension "d190" = 168.7
  dimension "d191" = 5
  dimension "d192" = 5
  dimension "d193" = 5
  dimension "d194" = 5
  dimension "d195" = 25
  dimension "d196" = 23
  dimension "d197" = 25
  dimension "d198" = 23
  constraint coincident L0.start L18.end
  constraint coincident L5.end L7.start
  constraint coincident L6.end L18.start
  constraint coincident L5.start L6.start
  constraint perpendicular L15 L54
  constraint parallel L41 L54
  constraint parallel L12 L15
  constraint coincident P0 L2
  constraint coincident P0 L21
  constraint coincident P0 L8.end
  constraint perpendicular L20 L40
  constraint parallel L40 L43
  constraint parallel L1 L20
  constraint coincident P4 L38
  constraint coincident P4 L19
  constraint coincident P4 L16.end
  constraint perpendicular L27 L34
  constraint parallel L33 L34
  constraint parallel L27 L35
  constraint coincident P1 L26
  constraint coincident P1 L29
  constraint coincident P1 L32.start
  constraint perpendicular L58 L60
  constraint parallel L59 L60
  constraint parallel L48 L58
  constraint coincident P2 L36
  constraint coincident P2 L30
  constraint coincident P2 L25.end
  constraint horizontal L62
  constraint vertical L63
  constraint horizontal L64
  constraint vertical L65
  constraint horizontal L66
  constraint vertical L67
  constraint horizontal L68
  constraint vertical L69
  constraint horizontal L70
  constraint vertical L71
  constraint horizontal L72
  constraint vertical L73
  constraint horizontal L74
  constraint vertical L75
  constraint horizontal L76
  constraint vertical L77
  constraint horizontal L78
  constraint vertical L79
  constraint horizontal L80
  constraint vertical L81
  constraint horizontal L82
  constraint vertical L83
  constraint horizontal L84
  constraint vertical L85
  constraint horizontal L86
  constraint vertical L87
  constraint horizontal L88
  constraint vertical L89
  constraint horizontal L90
  constraint vertical L91
  constraint horizontal L92
  constraint vertical L93
  measures "d115" distance of L51.end L6.end
  measures "d116" distance of L32.end L6.end
  measures "d117" distance of L5.start L16.start
  measures "d118" distance of L5.start L10.start
  measures "d119" distance of L5.end L8.start
  measures "d120" distance of L5.end L13.start
  measures "d121" distance of L25.start L11.start
  measures "d122" distance of L2.end L12.start
  measures "d123" distance of L2.end L15.start
  measures "d124" distance of L1.start L20.end
  measures "d125" distance of L19.start L20.end
  measures "d126" distance of L26.end L29.end
  measures "d127" distance of L27.start L26.end
  measures "d128" distance of L36.end L30.end
  measures "d129" distance of L36.end L30.start
  measures "d134" distance of L3.start L3.end
  measures "d135" distance of L4.start L3.start
  measures "d138" distance of L49.start L11.start
  measures "d147" distance of L62.start L3.start
  measures "d188" distance of L62.start L62.end
  measures "d189" distance of L62.start L64.end
  measures "d190" distance of L17.end L68.end
  measures "d191" distance of L68.end L70.end
  measures "d192" distance of L68.end L72.end
  measures "d193" distance of L67.end L74.end
  measures "d194" distance of L67.end L76.end
  measures "d195" distance of L3.start L82.end
  measures "d196" distance of L3.start L84.end
  measures "d197" distance of L75.end L86.end
  measures "d198" distance of L75.end L88.end
extrude "Extrude10" add sketch "Sketch7" along normal blind 7 separate body contours L0 L31 L47 L55 L67 L77 | L0 L31 L55 L67 L76 L77 | L6 L31 L32 L34 L35 L37 L44 L51 L53 | L31 L47 L50 L55 L67 L68 L74 L75 L77 | L11 L14 L24 L25 L28 L31 L48 L49 L52 L56 L57 L59 | L0 L5 L7 L8 L9 L11 L12 L14 L15 L22 L24 L25 L31 L41 L45 L47 L48 L52 L54 L57 L58 L59 L60 L61 L68 L69 L70 L73 | L0 L47 L55 L75 | L0 L55 L75 L76 | L31 L62 L67 L76 L81 L89 | L1 L5 L6 L7 L16 L20 L23 L27 L31 L32 L33 L34 L35 L40 L43 L44 L47 L53 L68 L74 | L47 L50 L55 L75 | L0 L9 L17 L22 L31 L42 L64 L66 L69 L73 | L25 L48 L52 L59 | L25 L48 L52 L58 L59 L60 | L0 L47 L68 L71 L75 | L0 L71 L75 L78 L86 | L31 L62 L63 L64 L65 L66 L67 | L5 L6 L7 L10 L16 L20 L23 L40 L44 L46 | L32 L34 L35 L53 | L27 L32 L33 L34 L35 L53 | L47 L68 L75 | L0 L68 L69 L70 L71 L73 | L0 L69 L71 L72 L73 | L78 L81 L86 L87 L88 L89 | L4 L65 L66 L80 L82 | L80 L81 L83 L88 L90 L91 | L16 L20 L23 L40 | L1 L16 L20 L23 L40 L43 | L5 L7 L8 L11 L13 L15 L24 L39 L41 L45 L57 L61 | L78 L79 L84 L87 L92 L93 | L3 L69 L72 L79 L85 | L79 L80 L82 L83 L84 L85 | L3 L4 L17 L42 L66 L69 | L8 L12 L15 L41 L54 L61 | L8 L15 L41 L61 | L90 L91 L92 L93 makes body 2
extrude "Extrude13" cut sketch "Sketch7" along normal blind 3.5 contours L25 L48 L52 L59 | L25 L48 L52 L58 L59 L60 | L32 L34 L35 L53 | L27 L32 L33 L34 L35 L53 | L16 L20 L23 L40 | L1 L16 L20 L23 L40 L43 | L8 L12 L15 L41 L54 L61 | L8 L15 L41 L61 bodies 2
extrude "Extrude14" add sketch "Sketch1" along normal blind 9 separate body contours L19 L20 L22 A2 L25 A6 L28 L29 L30 L31 | L19 L20 A2 L23 L24 L30 L31 | L21 L22 L25 L26 A6 L28 L29 makes body 3
extrude "Extrude15" add sketch "Sketch1" along normal blind 5 contours L19 L20 A2 A4 | L19 L20 A2 A4 | L22 L25 A6 A8 | L22 L25 A6 A8 | A0 | A5 | A7 | A11 | A13 | A18 | A20 | A23 | A24 | A25 | A27 | A28 | A32 | A33 | A36 | A38 | A39 | A40 | A41 | A42 | A45 bodies 3 1
sketch "Sketch9" plane through (0, 0, 9) normal (0, 0, 1) x (-1, 0, 0)
extrude "Extrude16" add sketch "Sketch7" along normal blind 14 contours L0 L31 L47 L55 L67 L77 | L0 L31 L55 L67 L76 L77 | L31 L47 L50 L55 L67 L68 L74 L75 L77 | L0 L47 L55 L75 | L0 L55 L75 L76 | L31 L62 L67 L76 L81 L89 | L47 L50 L55 L75 | L0 L47 L68 L71 L75 | L0 L71 L75 L78 L86 | L31 L62 L63 L64 L65 L66 L67 | L47 L68 L75 | L0 L68 L69 L70 L71 L73 | L0 L69 L71 L72 L73 | L4 L65 L66 L80 L82 | L3 L69 L72 L79 L85 | L3 L4 L17 L42 L66 L69 bodies 2
extrude "Extrude17" cut sketch "Sketch7" along normal blind 7 contours L90 L91 L92 L93 bodies 2
fillet "Fillet3" radius 2 2 edges at (417.9, 183.85, 10.5) (632, 183.85, 10.5) on bodies 2
fillet "Fillet3" radius 2 2 edges at (417.9, 15.15, 10.5) (632, 15.15, 10.5) on bodies 2
fillet "Fillet3" radius 1 4 edges at (627, 178.85, 10.5) (422.9, 178.85, 10.5) (422.9, 20.15, 10.5) (627, 20.15, 10.5) on bodies 2
extrude "Extrude18" add sketch "Sketch4" along normal blind 3 contours L32 L33 L53 L54 L55 L56 | L32 L33 L55 L56 | L20 L21 L47 L50 | L20 L21 L47 L48 L49 L50 | L28 L29 L36 L37 | L28 L29 L35 L36 L37 L38 | L24 L25 L41 L42 L43 L44 | L24 L25 L41 L42 bodies 1
sketch "Sketch10" plane through (0, 0, 102) normal (0, 0, 1) x (-1, 0, 0)
  line L0 (-226.875, -206.375) -> (-226.875, -202.625)
  line L1 (-226.875, -202.625) -> (-223.125, -202.625)
  line L2 (-223.125, -202.625) -> (-223.125, -206.375)
  line L3 (-223.125, -206.375) -> (-226.875, -206.375)
  line L4 (-226.875, 1.625) -> (-226.875, 5.375)
  line L5 (-226.875, 5.375) -> (-223.125, 5.375)
  line L6 (-223.125, 5.375) -> (-223.125, 1.625)
  line L7 (-223.125, 1.625) -> (-226.875, 1.625)
  line L8 (1.625, -206.375) -> (1.625, -202.625)
  line L9 (1.625, -202.625) -> (5.375, -202.625)
  line L10 (5.375, -202.625) -> (5.375, -206.375)
  line L11 (5.375, -206.375) -> (1.625, -206.375)
  line L12 (1.625, 1.625) -> (1.625, 5.375)
  line L13 (1.625, 5.375) -> (5.375, 5.375)
  line L14 (5.375, 5.375) -> (5.375, 1.625)
  line L15 (5.375, 1.625) -> (1.625, 1.625)
  line L16 (0, -201) -> (-232, -201)
  line L17 (-232, -201) -> (-232, -208)
  line L18 (-232, -208) -> (7, -208)
  line L19 (7, -208) -> (7, 7)
  line L20 (7, 7) -> (-232, 7)
  line L21 (-232, 0) -> (0, 0)
  line L22 (0, 0) -> (0, -201)
  line L23 (7, -208) -> (7, -178)
  line L24 (0, -178) -> (7, -178)
  line L25 (7, 7) -> (7, -23)
  line L26 (7, -23) -> (0, -23)
  line L27 (-232, 7) -> (-232, 0)
  dimension "d213" = 30
  dimension "d214" = 30
  constraint coincident L18.end L19.start
  constraint coincident L19 L23.end
  constraint coincident L22 L24.start
  constraint perpendicular L23 L24
  constraint coincident L19.end L20.start
  constraint perpendicular L20 L25
  constraint coincident L22 L26.end
  constraint perpendicular L22 L26
  measures "d213" distance of L18.end L23.end
  measures "d214" distance of L19.end L25.end
extrude "Extrude19" cut sketch "Sketch10" against normal blind 88 contours L19 L22 L24 L26 bodies 1
fillet "Fillet5" radius 2 8 edges at (-7, -7, 51) (232, -7, 56.5) (239, -7, 5.5) (239, 208, 5.5) (232, 208, 56.5) (232, 201, 56.5) (232, 0, 56.5) (-7, 208, 51) on bodies 1 2
fillet "Fillet5" radius 2 3 edges at (393, 207, 3.5) (632, 207, 3.5) (632, -8, 3.5) on bodies 1 2
fillet "Fillet5" radius 2 1 edges at (393, -8, 3.5) on bodies 1 2
extrude "Extrude20" add sketch "Sketch1" along normal blind 3 contours A47 | A49 | A51 | A53 | A55 | A57 | A59 | A61 | A63 bodies 1
extrude "Extrude21" add sketch "Sketch10" against normal blind 33 contours L19 L22 L24 L26 bodies 1
sketch "Sketch11" plane through (0, 0, 0) normal (0, 0, -1) x (1, 0, 0)
  circle A0 centre (16, -180) radius 3.375
  circle A1 centre (116, -105) radius 3.375
  circle A2 centre (216, -30) radius 3.375
  circle A3 centre (16, -105) radius 3.375
  circle A4 centre (116, -180) radius 3.375
  circle A5 centre (216, -105) radius 3.375
  circle A6 centre (116, -30) radius 3.375
  circle A7 centre (16, -30) radius 3.375
  circle A8 centre (216, -180) radius 3.375
  arc A9 (-7, -206) -> (-5, -208) centre (-5, -206) ccw
  line L0 (-5, -208) -> (237, -208)
  arc A10 (237, -208) -> (239, -206) centre (237, -206) ccw
  line L1 (239, -206) -> (239, 5)
  arc A11 (239, 5) -> (237, 7) centre (237, 5) ccw
  line L2 (237, 7) -> (-5, 7)
  arc A12 (-5, 7) -> (-7, 5) centre (-5, 5) ccw
  line L3 (-7, 5) -> (-7, -206)
  line L4 (-5, -210) -> (237, -210)
  arc A13 (237, -210) -> (241, -206) centre (237, -206) ccw
  line L5 (241, -206) -> (241, 5)
  arc A14 (241, 5) -> (237, 9) centre (237, 5) ccw
  line L6 (237, 9) -> (-5, 9)
  arc A15 (-5, 9) -> (-9, 5) centre (-5, 5) ccw
  line L7 (-9, 5) -> (-9, -206)
  arc A16 (-9, -206) -> (-5, -210) centre (-5, -206) ccw
  dimension "d239" = 2
extrude "Extrude22" add sketch "Sketch11" against normal up to surface (9 mm away) contours L4 A13 L5 A14 L6 A15 L7 A16 bodies 1 3
fillet "Fillet4" radius 2 2 edges at (-3.5, 23, 14) (-3.5, 178, 14) on bodies 1
fillet "Fillet4" radius 2 2 edges at (-3.5, 23, 69) (-3.5, 178, 69) on bodies 1
hidden bodies 2
equation "d57 = 100 mm + 2 mm"
equation "d61 = 9 mm + 2 mm"
equation "d65 = 7 mm + 15 mm"
equation "d67 = 33 mm + 15 mm"
equation "d72 = 7 mm + 15 mm"
equation "d201 = 7 mm + 7 mm"
